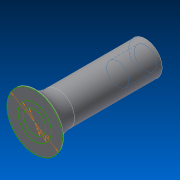
# Autodesk Inventor part: ssd standoff
Saved by Autodesk Inventor 2015 (Build 190159000, 159)
## iProperties
Created: 2017-03-27
Part Number: ssd standoff
Material: Generic
Document SubType Name: Modeling
Designer: ZigZagJoe
Density: 1 g/cm^3
Appearance: Default
Author: ZigZagJoe
Autodesk Inventor part; units mm, degrees
ref_plane "YZ Plane" through (0, 0, 0) normal (1, 0, 0) x (0, 1, 0)
ref_plane "XZ Plane" through (0, 0, 0) normal (0, 1, 0) x (-1, 0, 0)
ref_plane "XY Plane" through (0, 0, 0) normal (0, 0, 1) x (1, 0, 0)
sketch "Sketch1" plane through (0, 0, 0) normal (0, 1, 0) x (-1, 0, 0)
  circle A0 centre (0, 0) radius 2
  circle A1 centre (0, 0) radius 3
  circle A2 centre (0, 0) radius 5
  dimension "d0" = 4
  dimension "d1" = 6
  dimension "d2" = 10
  constraints: 3 centre point, 3 coincident
  measures "d0" diameter of A0
  measures "d1" diameter of A1
  measures "d2" diameter of A2
extrude "Extrusion1" add sketch "Sketch1" along normal blind 0.2 contours A1 | A2
extrude "Extrusion2" add sketch "Sketch1" along normal blind 20 contours A1
fillet "Fillet1" radius 5 1 edges at (3, 0.2, 0)
extrude "Extrusion3" add sketch "Sketch1" along normal blind 15 contours A0
body "Solid1"
